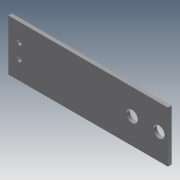
# Autodesk Inventor part: linac connector bar
Saved by Autodesk Inventor 2011 (Build 150239000, 239)
## iProperties
Created: 2011-12-28
Part Number: linac connector bar
Document SubType Name: Modeling
Designer: Matthew
Density: 1 g/cm^3
Author: Matthew
Autodesk Inventor part; units mm, degrees
ref_plane "YZ Plane" through (0, 0, 0) normal (1, 0, 0) x (0, 1, 0)
ref_plane "XZ Plane" through (0, 0, 0) normal (0, 1, 0) x (-1, 0, 0)
ref_plane "XY Plane" through (0, 0, 0) normal (0, 0, 1) x (1, 0, 0)
sketch "Sketch1" plane through (0, 0, 0) normal (0, 0, 1) x (1, 0, 0)
  line L0 (-34.9025, 5.6404) -> (104.7975, 5.6404)
  line L1 (104.7975, 5.6404) -> (104.7975, -26.3636)
  line L2 (104.7975, -26.3636) -> (-34.9025, -26.3636)
  line L3 (-34.9025, -26.3636) -> (-34.9025, 5.6404)
  point P0 (0, 0)
  dimension "d0" = 139.7
  dimension "d1" = 32.004
  constraints: 8 end point, 2 parallel, 1 horizontal, 1 perpendicular
  measures "d0" distance of L1.end L2.end
  measures "d1" distance of L0.end L1.end
extrude "Extrusion1" add sketch "Sketch1" along normal blind 3.175
sketch "Sketch2" plane through (-34.9025, 5.6404, 0) normal (0, 1, 0) x (1, 0, 0)
  line L0 (0, -3.175) -> (139.7, -3.175) projected
  line L1 (139.7, 0) -> (139.7, -3.175) projected
  line L2 (0, 0) -> (139.7, 0) projected
  line L3 (0, 0) -> (0, -3.175) projected
  point P0 (34.9025, 0)
extrude "Extrusion2" add sketch "Sketch2" along normal blind 12.7
sketch "Sketch3" plane through (0, 0, 3.175) normal (0, 0, 1) x (1, 0, 0)
  line L0 (104.7975, -26.3636) -> (-34.9025, -26.3636) projected
  line L1 (-34.9025, 18.3404) -> (-15.8525, 18.3404)
  line L2 (-15.8525, 18.3404) -> (-15.8525, -26.3636)
  line L3 (-15.8525, -26.3636) -> (-34.9025, -26.3636)
  line L4 (-34.9025, -26.3636) -> (-34.9025, 18.3404)
  line L5 (-34.9025, -4.0116) -> (-25.3775, -4.0116)
  line L6 (-25.3775, -4.0116) -> (-25.3775, 2.3384)
  line L7 (-25.3775, 2.3384) -> (-34.9025, 2.3384)
  line L8 (-34.9025, 2.3384) -> (-34.9025, -4.0116)
  line L9 (-25.3775, -4.0116) -> (-25.3775, -10.3616)
  circle A0 centre (-25.3775, 2.3384) radius 1.9812
  circle A1 centre (-25.3775, -10.3616) radius 1.9812
  point P0 (0, 0)
  dimension "d6" = 19.05
  dimension "d7" = 6.35
  dimension "d8" = 6.35
  dimension "d9" = 3.9624
  constraints: 18 end point, 5 parallel, 2 centre point, 2 coincident, 2 horizontal, 2 perpendicular, 1 midpoint, 1 point on line
  measures "d6" distance of L2.end L3.end
  measures "d7" distance of L6.end L5.end
  measures "d8" distance of L5.end L9.end
  measures "d9" diameter of A0
extrude "Extrusion3" cut sketch "Sketch3" against normal blind 12.7 contours A0 L6 L7 | L7 L6 A0 | A1
sketch "Sketch4" plane through (0, 0, 3.175) normal (0, 0, 1) x (1, 0, 0)
  line L0 (104.7975, 18.3404) -> (104.7975, -26.3636) projected
  line L1 (104.7975, -26.3636) -> (-34.9025, -26.3636) projected
  line L2 (104.7975, -4.0116) -> (96.7965, -4.0116)
  circle A0 centre (96.7965, -4.0116) radius 5.0038
  point P0 (0, 0)
  dimension "d12" = 8.001
  dimension "d13" = 10.0076
  constraints: 2 end point, 1 centre point, 1 coincident, 1 midpoint, 1 parallel
  measures "d12" distance of L2.start L2.end
  measures "d13" diameter of A0
extrude "Extrusion4" cut sketch "Sketch4" against normal blind 12.7
sketch "Sketch5" plane through (0, 0, 3.175) normal (0, 0, 1) x (1, 0, 0)
  circle A0 centre (96.7965, -4.0116) radius 5.0038 projected
  point P0 (0, 0)
extrude "Extrusion5" add sketch "Sketch5" against normal blind 3.175
sketch "Sketch6" plane through (0, 0, 3.175) normal (0, 0, 1) x (1, 0, 0)
  line L0 (104.7975, 18.3404) -> (104.7975, -26.3636) projected
  line L1 (104.7975, -26.3636) -> (-34.9025, -26.3636) projected
  line L2 (104.7975, -4.0116) -> (96.7975, -4.0116)
  circle A0 centre (96.7975, -4.0116) radius 5
  line L3 (103.3346, -4.0116) -> (73.3346, -4.0116)
  circle A1 centre (73.3346, -4.0116) radius 5
  point P0 (0, 0)
  dimension "d18" = 8
  dimension "d19" = 10
  dimension "d20" = 30
  constraints: 4 end point, 2 centre point, 2 coincident, 1 collinear, 1 midpoint, 1 parallel, 1 point on line
  measures "d18" distance of L2.start L2.end
  measures "d19" diameter of A0
  measures "d20" distance of L3.start L3.end
extrude "Extrusion6" cut sketch "Sketch6" against normal blind 3.175
body "Solid1"
